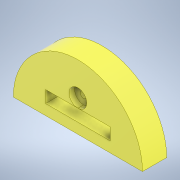
# Autodesk Inventor part: dRingHolder
Saved by Autodesk Inventor 2021.1 (Build 251245000, 245)
## iProperties
Created: 2020-09-12
Part Number: dRingHolder
Material: PBT Plastic
Document SubType Name: Modeling
Designer: robst
Density: 1.31 g/cm^3
Appearance: Smooth - Yellow
Author: robst
Autodesk Inventor part; units mm, degrees
ref_plane "YZ Plane" through (0, 0, 0) normal (1, 0, 0) x (0, 1, 0)
ref_plane "XZ Plane" through (0, 0, 0) normal (0, 1, 0) x (-1, 0, 0)
ref_plane "XY Plane" through (0, 0, 0) normal (0, 0, 1) x (1, 0, 0)
sketch "Sketch2" plane through (0, 0, 0) normal (0, 0, 1) x (1, 0, 0)
  arc A0 (31.75, 0) -> (-31.75, 0) centre (0, 0) ccw
  arc A1 (41.275, 0) -> (-41.275, 0) centre (0, 0) ccw
  line L0 (-41.275, 0) -> (-31.75, 0)
  line L1 (31.75, 0) -> (41.275, 0)
  arc A2 (50.8, 0) -> (-50.8, 0) centre (0, 0) ccw
  line L2 (-50.8, 0) -> (-41.275, 0)
  line L3 (41.275, 0) -> (50.8, 0)
  line L4 (-31.75, 0) -> (31.75, 0)
  line L5 (0, 0) -> (0, 31.75) construction
  line L6 (0, 8.255) -> (25.4, 8.255)
  line L7 (25.4, 8.255) -> (25.4, 17.78)
  line L8 (25.4, 17.78) -> (0, 17.78)
  line L9 (0, 17.78) -> (-25.4, 17.78)
  line L10 (-25.4, 17.78) -> (-25.4, 8.255)
  line L11 (-25.4, 8.255) -> (0, 8.255)
  dimension "d2" = 63.5
  dimension "d3" = 9.525
  dimension "d4" = 9.525
  dimension "d5" = 25.4
  dimension "d6" = 8.255
  dimension "d7" = 9.525
  constraints: 24 end point, 7 point on circle, 7 point on line, 3 centre point, 3 coincident, 3 collinear, 3 horizontal, 3 perpendicular
  measures "d2" diameter of A0
  measures "d3" radial gap between concentric circles of A1 A0
  measures "d4" radial gap between concentric circles of A2 A1
  measures "d5" distance from line of L7.end L5
  measures "d6" distance of L6.start point (0, 0)
  measures "d7" distance of L9.end L10.end
extrude "Extrusion1" add sketch "Sketch2" along normal blind 6.35
extrude "Extrusion2" add sketch "Sketch2" against normal blind 12.7 contours L4 A0 | A1 L2 A2 L3
sketch "Sketch5" plane through (0, 0, 6.35) normal (0, 0, 1) x (1, 0, 0)
  line L0 (-25.4, 17.78) -> (25.4, 17.78) projected
  arc A0 (31.75, 0) -> (-31.75, 0) centre (0, 0) ccw projected
  line L1 (0, 17.78) -> (0, 31.75) construction
  arc A1 (31.75, 0) -> (-31.75, 0) centre (0, 0) ccw construction
  point P0 (0, 24.765)
  constraints: 2 end point, 2 midpoint, 2 point on circle
hole "Hole2" at (0, 24.765, 6.35) direction (0, 0, -1) diameter 5.1054 end through all counterbore diameter 13.97 counterbore depth 4.445 clearance for "Socket Head Cap Screw" size "#10" standard "Ansi Unified Screw Threads"
equation "\"d2\" = insideDiameterOfRing"
equation "\"d3\" = innerRingWidth"
equation "\"d4\" = outerRingWidth"
equation "\"d5\" = halfWidthForPryBar"
equation "\"d6\" = distanceFromEdgeToPryBar"
equation "\"d7\" = depthForPryBar"
equation "\"d8\" = topPartHeight"
equation "\"d10\" = lowerPartHeight"
equation "\"insideDiameterOfRing\" = 63.5"
equation "\"wallThicknessOfRing\" = 9.525"
equation "\"outsideDiameterOfRing\" = insideDiameterOfRing + 2 * wallThicknessOfRing"
equation "\"widthForPryBar\" = 50.8"
equation "\"outerRingWidth\" = 9.525"
equation "\"innerRingWidth\" = 9.525"
equation "\"halfWidthForPryBar\" = 0.5 * widthForPryBar"
equation "\"distanceFromEdgeToPryBar\" = 8.255"
equation "\"totalHeightOfPart\" = 19.05"
equation "\"topPartHeight\" = 6.35"
equation "\"lowerPartHeight\" = totalHeightOfPart - topPartHeight"
equation "\"depthForPryBar\" = 9.525"
body "Solid1"
